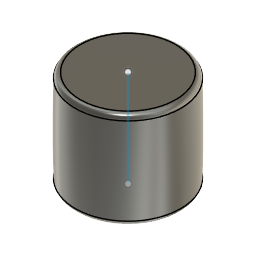
fork-upper-crown0-type-af7mm-fox34-miran (Autodesk Fusion 360 archive; units mm, degrees)
design "34 crown"
part number: 2026-09-07-17-33-09-663
Autodesk Fusion 360 part; units mm, degrees
sketch "Sketch1" plane through (0, 0, 0) normal (0, 1, 0) x (1, 0, 0)
  line L0 (361.5532, -44.2022) -> (361.5532, -6.2022)
  line L1 (361.5532, -25.2022) -> (382.5532, -25.2022) construction
  line L2 (361.5532, -42.2022) -> (382.3032, -42.2022) construction
  line L3 (361.5532, -8.2022) -> (382.3032, -8.2022) construction
  line L4 (361.5532, -44.2022) -> (380.3024, -44.2022)
  line L5 (361.5532, -6.2022) -> (380.3024, -6.2022)
  arc A0 (382.3015, -42.2612) -> (382.3015, -8.1432) centre (-195.5718, -25.2022) ccw
  arc A1 (380.3024, -44.2022) -> (382.3015, -42.2612) centre (380.3024, -42.2022) ccw
  arc A2 (382.3015, -8.1432) -> (380.3024, -6.2022) centre (380.3024, -8.2022) ccw
  dimension "d1" = 38
  dimension "d2" = 21
  dimension "d3" = 20.75
  dimension "d4" = 2
  dimension "d5" = 2
  dimension "d6" = 2
  constraint vertical L0
  constraint midpoint L0 L1.start
  constraint perpendicular L0 L1
  constraint coincident L0 L2.start
  constraint perpendicular L0 L2
  constraint symmetric L1 L2.start L3.start
  constraint symmetric L1 L2.end L3.end
  constraint coincident L2.end A0
  constraint coincident L1.end A0
  constraint coincident L3.end A0
  constraint perpendicular L0 L4
  constraint perpendicular L0 L5
  constraint tangent A0 A1
  constraint tangent L4 A1
  constraint tangent A0 A2
  constraint tangent L5 A2
  measures "d1" distance of L0.start L0.end
  measures "d2" distance of L1.start L1.end
  measures "d3" distance of L2.start L2.end
  measures "d4" distance of L0.start L2
  measures "d5" radius of A1
  measures "d6" radius of A2
revolve "Revolve1" add sketch "Sketch1" angle 360 about axis through (361.5532, 0, 44.2022) along (0, 0, -1)
